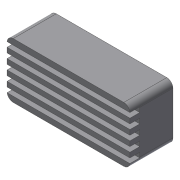
# Autodesk Inventor part: Victor
Saved by Autodesk Inventor 2016 (Build 200138000, 138)
## iProperties
Created: 2016-01-27
Part Number: Victor
Material: Generic
Document SubType Name: Modeling
Designer: PrashantBIA
Density: 1 g/cm^3
Appearance: Default
Author: PrashantBIA
Autodesk Inventor part; units mm, degrees
ref_plane "YZ Plane" through (0, 0, 0) normal (1, 0, 0) x (0, 1, 0)
ref_plane "XZ Plane" through (0, 0, 0) normal (0, 1, 0) x (-1, 0, 0)
ref_plane "XY Plane" through (0, 0, 0) normal (0, 0, 1) x (1, 0, 0)
sketch "Sketch1" plane through (0, 0, 0) normal (0, 0, 1) x (1, 0, 0)
  line L0 (0, 0) -> (63.5, 0)
  line L1 (63.5, 0) -> (63.5, 28.575)
  line L2 (63.5, 28.575) -> (0, 28.575)
  line L3 (0, 28.575) -> (0, 0)
  dimension "d0" = 63.5
  dimension "d1" = 28.575
  constraints: 8 end point, 2 parallel, 1 horizontal, 1 perpendicular
  measures "d0" distance of L1.end L2.end
  measures "d1" distance of L0.end L1.end
extrude "Extrusion1" add sketch "Sketch1" along normal blind 22.225
fillet "Fillet1" radius 3.175 4 edges at (63.5, 28.575, 11.1125) (63.5, 0, 11.1125) (0, 0, 11.1125) (0, 28.575, 11.1125)
sketch "Sketch2" plane through (0, 0, 22.225) normal (0, 0, 1) x (1, 0, 0)
  line L0 (63.5, 3.175) -> (63.5, 25.4) projected
  line L1 (0, 25.6349) -> (63.5, 25.6349)
  line L2 (63.5, 25.6349) -> (63.5, 23.0949)
  line L3 (63.5, 23.0949) -> (0, 23.0949)
  line L4 (0, 23.0949) -> (0, 25.6349)
  line L5 (0, 20.5549) -> (63.5, 20.5549)
  line L6 (63.5, 20.5549) -> (63.5, 18.0149)
  line L7 (63.5, 18.0149) -> (0, 18.0149)
  line L8 (0, 18.0149) -> (0, 20.5549)
  line L9 (0, 15.4749) -> (63.5, 15.4749)
  line L10 (63.5, 15.4749) -> (63.5, 12.9349)
  line L11 (63.5, 12.9349) -> (0, 12.9349)
  line L12 (0, 12.9349) -> (0, 15.4749)
  line L13 (0, 10.3949) -> (63.5, 10.3949)
  line L14 (63.5, 10.3949) -> (63.5, 7.8549)
  line L15 (63.5, 7.8549) -> (0, 7.8549)
  line L16 (0, 7.8549) -> (0, 10.3949)
  line L17 (0, 5.3149) -> (63.5, 5.3149)
  line L18 (63.5, 5.3149) -> (63.5, 2.7749)
  line L19 (63.5, 2.7749) -> (0, 2.7749)
  line L20 (0, 2.7749) -> (0, 5.3149)
  point P0 (0, 0)
  dimension "d5" = 2.54
  dimension "d8" = 5.08
  constraints: 40 end point, 2 parallel, 1 collinear, 1 horizontal, 1 perpendicular, 1 point on line, 1 vertical, 31 other
  measures "d5" distance of L3.end L1.start
  measures "d8" distance of L1.start L5.start
extrude "Extrusion2" cut sketch "Sketch2" against normal blind 5.08
body "Solid1"
